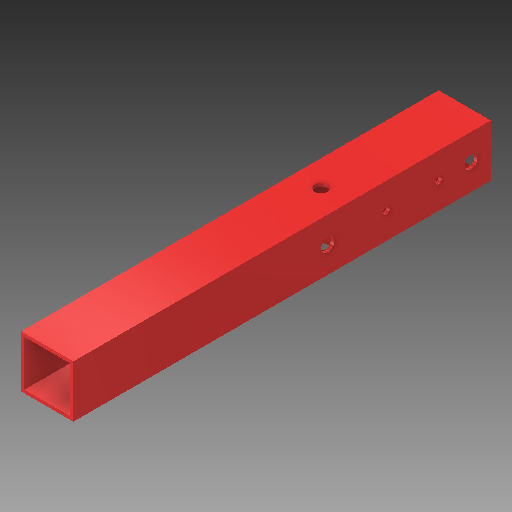
# Autodesk Inventor part: Upright
Saved by Autodesk Inventor 2017 (Build 210142000, 142)
## iProperties
Created: 2017-01-16
Part Number: Upright
Material: Aluminum 6061
Document SubType Name: Modeling
Designer: Ben
Density: 2.7 g/cm^3
Appearance: Light Red
Mass: 81.9279 g
Surface Area: 388.473 cm^2
Volume: 30.3437 cm^3
Author: Ben
Autodesk Inventor part; units mm, degrees
ref_plane "YZ Plane" through (0, 0, 0) normal (1, 0, 0) x (0, 1, 0)
ref_plane "XZ Plane" through (0, 0, 0) normal (0, 1, 0) x (-1, 0, 0)
ref_plane "XY Plane" through (0, 0, 0) normal (0, 0, 1) x (1, 0, 0)
sketch "Sketch1" plane through (0, 0, 0) normal (0, 0, 1) x (1, 0, 0)
  line L0 (0, 0) -> (-11.1125, 0) construction
  line L1 (0, 0) -> (0, 11.1125) construction
  line L2 (-11.1125, 11.1125) -> (11.1125, 11.1125)
  line L3 (11.1125, 11.1125) -> (11.1125, -11.1125)
  line L4 (11.1125, -11.1125) -> (-11.1125, -11.1125)
  line L5 (-11.1125, -11.1125) -> (-11.1125, 11.1125)
  line L6 (-12.7, 12.7) -> (12.7, 12.7)
  line L7 (12.7, 12.7) -> (12.7, -12.7)
  line L8 (12.7, -12.7) -> (-12.7, -12.7)
  line L9 (-12.7, -12.7) -> (-12.7, 12.7)
  line L10 (-11.1125, 0) -> (-12.7, 0) construction
  line L11 (0, 11.1125) -> (0, 12.7) construction
  dimension "d0" = 25.4
  dimension "d1" = 1.5875
  constraints: 24 end point, 4 horizontal, 4 midpoint, 4 parallel, 4 perpendicular, 2 vertical
  measures "d0" distance of L8.end L6.start
  measures "d1" distance of L1.end L11.end
extrude "Extrusion1" add sketch "Sketch1" along normal blind 203.2
sketch "Sketch2" plane through (-12.7, 12.7, 0) normal (0, 1, 0) x (1, 0, 0)
  line L0 (12.7, 0) -> (12.7, -203.2) construction
  line L1 (25.4, 0) -> (25.4, -203.2) construction
  circle A0 centre (12.7, -69.85) radius 3.175
  dimension "d4" = 6.35
  dimension "d5" = 69.85
  constraints: 2 end point, 1 centre point, 1 parallel, 1 point on line
  measures "d4" diameter of A0
  measures "d5" distance of A0.centre L0.start
extrude "Extrusion2" cut sketch "Sketch2" against normal through all
sketch "Sketch3" plane through (12.7, -12.7, 0) normal (1, 0, 0) x (0, 0, -1)
  line L0 (0, 12.7) -> (-203.2, 12.7) construction
  line L1 (0, 23.8125) -> (-203.2, 23.8125) construction
  circle A0 centre (-79.375, 12.7) radius 3.175
  circle A1 centre (-9.525, 12.7) radius 3.175
  line L2 (0, 25.4) -> (0, 0) projected
  line L3 (-38.1, 23.8125) -> (-38.1, 12.7) construction
  circle A2 centre (-50.8, 12.7) radius 1.5875
  circle A3 centre (-25.4, 12.7) radius 1.5875
  dimension "d8" = 6.35
  dimension "d9" = 79.375
  dimension "d12" = 6.35
  dimension "d13" = 9.525
  dimension "d22" = 3.175
  dimension "d23" = 25.4
  dimension "d24" = 38.1
  constraints: 6 point on line, 4 centre point, 4 end point, 1 equal radius, 1 parallel, 1 perpendicular, 1 other
  measures "d8" diameter of A0
  measures "d9" distance of L0.start A0.centre
  measures "d12" diameter of A1
  measures "d13" distance from line of L2 A1.centre
  measures "d22" diameter of A2
  measures "d23" distance of A3.centre A2.centre
  measures "d24" distance between parallel lines of L2 L3
extrude "Extrusion3" cut sketch "Sketch3" against normal through all
body "Solid1"
